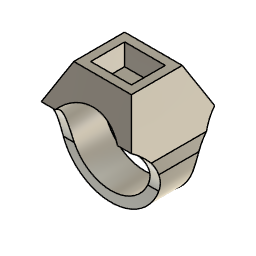
14 (Autodesk Fusion 360 design; units mm, degrees)
Autodesk Fusion 360 part; units mm, degrees
sketch "草图1" plane through (0, 0, 0) normal (0, 1, 0) x (1, 0, 0)
  circle A0 centre (0, 0) radius 12
  line L0 (-8.5, -18) -> (8.5, -18)
  line L1 (8.5, -18) -> (15, -4.0607)
  line L2 (-8.5, -18) -> (-15, -4.0607)
  line L3 (0, -38) -> (0, 21) construction
  line L4 (-34, 0) -> (39, 0) construction
  line L5 (-15, 0) -> (-15, -4.0607)
  line L6 (15, 0) -> (15, -4.0607)
  arc A1 (15, 0) -> (-15, 0) centre (0, 0) ccw
  dimension "d1" = 30
  dimension "d2" = 24
  dimension "d3" = 18
  dimension "d4" = 65
  dimension "d5" = 17
  constraint coincident A0.centre A1.centre
  constraint concentric A0 A1
  constraint horizontal L0
  constraint vertical L3
  constraint horizontal L4
  constraint symmetric L1 L2 L3
  constraint coincident L4 L5.start
  constraint perpendicular L4 L5
  constraint coincident L4 L6.start
  constraint perpendicular L4 L6
  measures "d1" diameter of A1
  measures "d2" diameter of A0
  measures "d3" distance of A0.centre L0
  measures "d4" angle of L0 L2
  measures "d5" distance of L0.start L0.end
extrude "拉伸1" add sketch "草图1" along normal mid plane 30 makes body 1
sketch "草图2" plane through (0, 0, 18) normal (0, 0, 1) x (-1, 0, 0)
  line L0 (-8.5, 15) -> (-8.5, -15)
  line L1 (-8.5, -15) -> (8.5, -15)
  line L2 (8.5, -15) -> (8.5, 15)
  line L3 (8.5, 15) -> (-8.5, 15)
  line L4 (-8.5, 7.5) -> (8.5, 7.5)
  line L5 (8.5, 7.5) -> (8.5, -7.5)
  line L6 (8.5, -7.5) -> (-8.5, -7.5)
  line L7 (-8.5, -7.5) -> (-8.5, 7.5)
  line L8 (-8.5, 7.5) -> (8.5, -7.5) construction
  line L9 (8.5, 7.5) -> (-8.5, -7.5) construction
  dimension "d8" = 15
  constraint horizontal L4
  constraint perpendicular L4 L5
  constraint parallel L4 L6
  constraint parallel L5 L7
  constraint coincident L8 origin
  constraint coincident L9 origin
  constraint coincident L0 L4.start
  measures "d8" distance of L4.start L6.end
sketch "草图3" plane through (-15, 0, 0) normal (-1, 0, 0) x (0, -1, 0)
  line L0 (15, 4.0607) -> (-15, 4.0607)
  line L1 (-15, 4.0607) -> (-15, 0)
  line L2 (-15, 0) -> (15, 0)
  line L3 (15, 0) -> (15, 4.0607)
  line L4 (-5, -15) -> (5, -15)
  line L5 (5, -15) -> (5, -5.1421)
  line L6 (-5, -15) -> (-5, -5.1421)
  line L7 (-15, 18) -> (15, 18)
  line L8 (15, 18) -> (15, -15)
  line L9 (15, -15) -> (-15, -15)
  line L10 (-15, -15) -> (-15, 18)
  arc A0 (-5, -5.1421) -> (-15, 9) centre (-20, -5.1421) ccw
  arc A1 (15, 9) -> (5, -5.1421) centre (20, -5.1421) ccw
  line L11 (0, 21) -> (0, -19) construction
  point P0 (15, 18)
  dimension "d9" = 9
  dimension "d10" = 10
  dimension "d11" = 15
  constraint parallel L2 L4
  constraint perpendicular L4 L5
  constraint perpendicular L4 L6
  constraint horizontal L7
  constraint vertical L8
  constraint horizontal L9
  constraint vertical L10
  constraint coincident L10 A0.end
  constraint coincident L8 A1.start
  constraint perpendicular L7 L11
  constraint symmetric A0 A1 L11
  constraint collinear L4 L9
  constraint tangent L5 A1
  measures "d9" distance of A1.start P0
  measures "d10" distance of L4.start L4.end
  measures "d11" radius of A1
extrude "拉伸2" cut sketch "草图3" against normal blind 48 contours L0 L2 L3 L8 A1 | L0 L8 A1 | L2 L5 L8 L9 A1 | L0 L1 L2 L10 A0 | L0 L10 A0 | L2 L6 L9 L10 A0 bodies 1
sketch "草图4" plane through (-15, 0, 0) normal (-1, 0, 0) x (0, -1, 0)
  arc A0 (-5.9089, 0) -> (-8.1548, 4.0607) centre (-20, -5.1421) ccw
  line L0 (-5.9089, 0) -> (5.9089, 0)
  arc A1 (8.1548, 4.0607) -> (5.9089, 0) centre (20, -5.1421) ccw
  line L1 (8.1548, 4.0607) -> (-8.1548, 4.0607)
  line L2 (-15, 18) -> (15, 18)
  line L3 (15, 18) -> (15, 9)
  line L4 (15, 9) -> (-15, 9)
  line L5 (-15, 9) -> (-15, 18)
  line L6 (0, 23) -> (0, -21) construction
  line L7 (-7.5, 18) -> (-17.1867, -2.7731)
  line L8 (-17.1867, -2.7731) -> (17.1867, -2.7731)
  line L9 (17.1867, -2.7731) -> (7.5, 18)
  line L10 (-7.5, 18) -> (7.5, 18)
  line L11 (-15, 18) -> (17.1867, 18)
  line L12 (17.1867, 18) -> (17.1867, -2.7731)
  line L13 (17.1867, -2.7731) -> (-15, -2.7731)
  line L14 (-15, -2.7731) -> (-15, 18)
  dimension "d14" = 15
  dimension "d15" = 65
  dimension "d16" = 65
  constraint horizontal L2
  constraint vertical L3
  constraint horizontal L4
  constraint vertical L5
  constraint perpendicular L0 L6
  constraint coincident L2 L7.start
  constraint parallel L2 L8
  constraint coincident L2 L9.end
  constraint symmetric L6 L7.start L9.end
  constraint horizontal L11
  constraint vertical L12
  constraint horizontal L13
  constraint vertical L14
  measures "d14" distance of L7.start L9.end
  measures "d15" angle of L2 L7
  measures "d16" angle of L2 L9
extrude "拉伸3" cut sketch "草图4" against normal blind 39 contours L2 L4 L5 L7 L11 L14 | L4 L7 L14 | L2 L3 L4 L9 L11 | L3 L4 L9 L11 L12 bodies 1
sketch "草图5" plane through (0, 0, 18) normal (0, 0, 1) x (-1, 0, 0)
  line L0 (6, -5) -> (-6, -5)
  line L1 (-6, -5) -> (-6, 5)
  line L2 (-6, 5) -> (6, 5)
  line L3 (6, 5) -> (6, -5)
  line L4 (6, -5) -> (-6, 5) construction
  line L5 (-6, -5) -> (6, 5) construction
  dimension "d19" = 10
  dimension "d20" = 12
  constraint horizontal L0
  constraint perpendicular L0 L1
  constraint parallel L0 L2
  constraint parallel L1 L3
  constraint coincident L4 origin
  constraint coincident L5 origin
  measures "d19" distance of L0.start L2.end
  measures "d20" distance of L1.end L2.end
extrude "拉伸4" cut sketch "草图5" against normal blind 5 bodies 1
sketch "草图6" plane through (6, 0, 0) normal (-1, 0, 0) x (0, -1, 0)
  line L0 (5, 18) -> (-5, 18)
  line L1 (-5, 18) -> (-5, 13)
  line L2 (-5, 13) -> (5, 13)
  line L3 (5, 13) -> (5, 18)
  line L4 (-5, 18) -> (-5, 13)
  line L5 (5, 13) -> (5, 18)
  line L6 (-5, 18) -> (-3.6603, 13)
  line L7 (5, 18) -> (3.6603, 13)
  line L8 (5, 13) -> (3.6603, 13)
  line L9 (-3.6603, 13) -> (-5, 13)
  line L10 (0, 22) -> (0, 5.5125) construction
  dimension "d23" = 30
  constraint coincident L0.end L1.start
  constraint coincident L1.end L2.start
  constraint coincident L2.end L3.start
  constraint coincident L0.start L3.end
  constraint coincident L2 L6.end
  constraint coincident L2 L7.end
  constraint vertical L10
  constraint symmetric L6 L7 L10
  measures "d23" angle of L6 L7
extrude "拉伸5" add sketch "草图6" along normal blind 12 separate body contours L2 L3 L5 L7 L8 | L1 L2 L4 L6 L9 makes body 2 at (2, 4.5534, 16.3333) makes body 3 at (-2, -4.1068, 14.6667)
sketch "草图7" plane through (0, -5, 0) normal (0, 1, 0) x (-1, 0, 0)
  line L0 (6, 18) -> (-6, 18)
  line L1 (-6, 18) -> (-6, 13)
  line L2 (-6, 13) -> (6, 13)
  line L3 (6, 13) -> (6, 18)
  line L4 (-6, 18) -> (-6, 13)
  line L5 (0, 24) -> (0, 4) construction
  line L6 (6, 18) -> (6, 13)
  line L7 (-6, 13) -> (6, 13)
  line L8 (6, 18) -> (4.6603, 13)
  line L9 (-6, 18) -> (-4.6603, 13)
  dimension "d26" = 30
  constraint coincident L0.end L1.start
  constraint coincident L1.end L2.start
  constraint perpendicular L2 L5
  constraint coincident L0.start L3.end
  constraint coincident L2.end L3.start
  constraint coincident L2 L8.end
  constraint coincident L2 L9.end
  constraint symmetric L5 L8 L9
  measures "d26" angle of L8 L9
extrude "拉伸6" add sketch "草图7" along normal blind 10 separate body contours L2 L3 L6 L7 L8 | L1 L2 L4 L7 L9 makes body 4 at (5.5534, -1.6667, 16.3333) makes body 5 at (-5.5534, -1.6667, 16.3333)
combine "合并1" operation add target body 1 tool bodies 2 3 5 4
